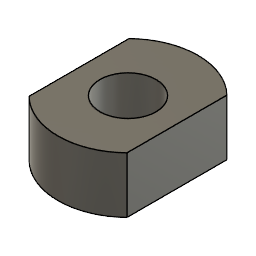
P1 (Autodesk Fusion 360 design; units mm, degrees)
part number: 2026-08-20-08-42-54-312
Autodesk Fusion 360 part; units mm, degrees
sketch "Sketch1" plane through (0, 0, 0) normal (0, 1, 0) x (1, 0, 0)
  circle A0 centre (0, 0) radius 20
  line L0 (-35, 35.7071) -> (-35, -35.7071)
  line L1 (0, 0) -> (0, 70.7339) construction
  line L2 (35, 35.7071) -> (35, -35.7071)
  arc A1 (-35, -35.7071) -> (35, -35.7071) centre (0, 0) ccw
  arc A2 (35, 35.7071) -> (-35, 35.7071) centre (0, 0) ccw
  dimension "d1" = 40
  dimension "d2" = 100
  dimension "d3" = 70
  dimension "d6" = 35
  constraint coincident A0.centre L1.start
  constraint vertical L0
  constraint vertical L1
  constraint concentric A1 A2
  measures "d1" diameter of A0
  measures "d2" diameter of A1
  measures "d3" distance of L0 L2
  measures "d6" distance of A0.centre L2
extrude "Extrude1" add sketch "Sketch1" along normal mid plane 40
